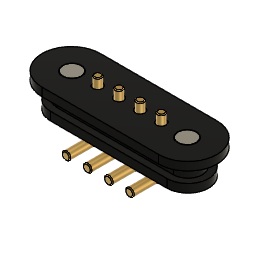
5358 Mag Connector (4-pin, Right Angle, Pins) (Autodesk Fusion 360 design; units mm, degrees)
Autodesk Fusion 360 part; units mm, degrees
sketch "Profile" plane through (0, 0, 0) normal (0, 0, 1) x (1, 0, 0)
  line L0 (0, 3.5) -> (0, -3.5) construction
  circle A0 centre (-6.91, 0) radius 1.125
  circle A1 centre (-3.81, 0) radius 0.45
  circle A2 centre (-1.27, 0) radius 0.45
  circle A3 centre (1.27, 0) radius 0.45
  circle A4 centre (6.91, 0) radius 1.125
  circle A5 centre (-3.81, 0) radius 0.5
  circle A6 centre (-3.81, 0) radius 0.9
  circle A7 centre (-1.27, 0) radius 0.5
  circle A8 centre (-1.27, 0) radius 0.9
  circle A9 centre (1.27, 0) radius 0.5
  circle A10 centre (1.27, 0) radius 0.9
  circle A11 centre (-3.81, 0) radius 0.575
  circle A12 centre (-1.27, 0) radius 0.575
  circle A13 centre (1.27, 0) radius 0.575
  line L1 (-10.5, 0) -> (10.5, 0) construction
  line L2 (-7, 1.725) -> (-7, -1.725) construction
  line L3 (-7, 2.5) -> (-7, -2.5) construction
  line L4 (-7, 3.5) -> (-7, -3.5) construction
  arc A14 (-7, 3.5) -> (-7, -3.5) centre (-7, 0) ccw
  arc A15 (-7, 1.725) -> (-7, -1.725) centre (-7, 0) ccw
  arc A16 (-7, 2.5) -> (-7, -2.5) centre (-7, 0) ccw
  line L5 (0, 3.5) -> (-7, 3.5)
  line L6 (0, -3.5) -> (-7, -3.5)
  line L7 (-7, 2.5) -> (0, 2.5)
  line L8 (-7, 1.725) -> (0, 1.725)
  line L9 (-7, -1.725) -> (0, -1.725)
  line L10 (-7, -2.5) -> (0, -2.5)
  circle A17 centre (3.81, 0) radius 0.45
  circle A18 centre (3.81, 0) radius 0.5
  circle A19 centre (3.81, 0) radius 0.9
  circle A20 centre (3.81, 0) radius 0.575
  line L11 (7, 1.725) -> (0, 1.725)
  line L12 (7, 2.5) -> (0, 2.5)
  line L13 (0, 3.5) -> (7, 3.5)
  arc A21 (7, -3.5) -> (7, 3.5) centre (7, 0) ccw
  arc A22 (7, -2.5) -> (7, 2.5) centre (7, 0) ccw
  arc A23 (7, -1.725) -> (7, 1.725) centre (7, 0) ccw
  line L14 (7, -1.725) -> (0, -1.725)
  line L15 (7, -2.5) -> (0, -2.5)
  line L16 (0, -3.5) -> (7, -3.5)
  line L17 (1, 3.375) -> (-1, 3.375)
  line L18 (1, 3.375) -> (1.875, 2.5)
  line L19 (-1, 3.375) -> (-1.875, 2.5)
  line L20 (1.25, 2.5) -> (1.25, 1.9)
  line L21 (1.25, 1.9) -> (-1.25, 1.9)
  line L22 (-1.25, 1.9) -> (-1.25, 2.5)
  dimension "d1" = 2.25
  dimension "d10" = 0.9
  dimension "d11" = 3.1
  dimension "d16" = 2.54
  dimension "d17" = 0
  dimension "d19" = 1
  dimension "d20" = 1.8
  dimension "d45" = 1.15
  dimension "d91" = 13.82
  dimension "d92" = 21
  dimension "d93" = 3.45
  dimension "d94" = 5
  dimension "d95" = 7
  dimension "d104" = 2
  dimension "d105" = 3.75
  dimension "d107" = 45
  dimension "d108" = 0.6
  dimension "d109" = 2.5
  constraint vertical L0
  constraint symmetric L0 A0 A4
  constraint concentric A1 A5
  constraint concentric A1 A6
  constraint midpoint origin L0
  constraint concentric A6 A11
  constraint horizontal L1
  constraint coincident A0.centre L1
  constraint coincident A1.centre L1
  constraint coincident L1 origin
  constraint midpoint L1 origin
  constraint perpendicular L1 L2
  constraint symmetric L1 L2.start L2.end
  constraint perpendicular L1 L3
  constraint symmetric L1 L3.start L3.end
  constraint vertical L4
  constraint symmetric L1 L4.start L4.end
  constraint midpoint L4 A14.centre
  constraint coincident L1.start A14
  constraint midpoint L2 A14.centre
  constraint midpoint L3 A14.centre
  constraint perpendicular L0 L5
  constraint perpendicular L0 L6
  constraint coincident L4.end A14.end
  constraint coincident A14 L4.start
  constraint collinear L2 L4
  constraint collinear L3 L4
  constraint coincident L0 L7.end
  constraint tangent A16 L7
  constraint coincident L0 L8.end
  constraint tangent A15 L8
  constraint coincident L0 L9.end
  constraint tangent A15 L9
  constraint coincident L0 L10.end
  constraint tangent A16 L10
  constraint symmetric L5.start L0 L13.start
  constraint symmetric L6.start L0 L16.start
  constraint symmetric L0 L2.start L11.start
  constraint symmetric L0 L2.end A23.start
  constraint symmetric L0 L3.start L12.start
  constraint symmetric L0 L3.end A22.start
  constraint symmetric L0 L4.start L13.end
  constraint symmetric L0 L4.end A21.start
  constraint symmetric L0 A14 A21
  constraint symmetric L0 A15 A23
  constraint symmetric L0 A16 A22
  constraint symmetric L0 L7.end L12.end
  constraint symmetric L0 L8.end L11.end
  constraint symmetric L0 L9.end L14.end
  constraint symmetric L0 L10.end L15.end
  constraint parallel L13 L17
  constraint symmetric L0 L17.start L17.end
  constraint coincident L12 L18.end
  constraint coincident L7 L19.end
  constraint symmetric L0 L18.end L19.end
  constraint coincident L12 L20.start
  constraint perpendicular L12 L20
  constraint perpendicular L20 L21
  constraint coincident L7 L22.end
  constraint perpendicular L7 L22
  constraint symmetric L0 L20.end L21.end
  measures "d1" diameter of A0
  measures "d10" diameter of A1
  measures "d11" distance of A0.centre A1.centre
  measures "d19" diameter of A5
  measures "d20" diameter of A6
  measures "d45" diameter of A11
  measures "d91" distance of A0.centre A4.centre
  measures "d92" distance of L1.start L1.end
  measures "d93" distance of L2.start L2.end
  measures "d94" distance of L3.start L3.end
  measures "d95" distance of L0.start L0.end
  measures "d104" distance of L17.start L17.end
  measures "d105" distance of L18.end L19.end
  measures "d107" angle of L17 L19
  measures "d108" distance of L20.start L20.end
  measures "d109" distance of L20.end L21.end
extrude "Extrude - Housing" add sketch "Profile" along normal blind 4 contours A15 L8 L9 L11 A23 L14 makes body 1
extrude "Extrude6" add sketch "Profile" against normal blind 1 from surface at 4 contours A14 L5 L6 L13 A21 L16 | A16 L7 L10 L12 A22 L15 L20 L21 L22 | L7 L12 L17 L18 L19 | L7 L12 L20 L21 L22 bodies 1
extrude "Extrude7" add sketch "Profile" against normal blind 0.65 from surface at 3 contours A16 L7 L10 L12 A22 L15 L20 L21 L22 | L7 L12 L20 L21 L22 bodies 1
extrude "Extrude8" add sketch "Profile" along normal blind 1 contours A16 L7 L10 L12 A22 L15 L20 L21 L22 | L7 L12 L20 L21 L22 bodies 1
extrude "Extrude - Housing Pin Clearance" add sketch "Profile" along normal up to surface (3.8 mm away) from surface at 0.2 contours A6 | A8 | A10 | A19 bodies 1
copy_body "Body->Comp1" bodies 1 removing the originals makes body 2 in component "Housing"
extrude "Extrude - Magnets" add sketch "Profile" along normal blind 4 separate body contours A0 | A4 makes body 3 at (-5.7906, -0.112, 1.3333) makes body 4 at (8.0336, -0.0561, 2.6667)
copy_body "Body->Comp2" bodies 3 removing the originals makes body 5 in component "Magnet"
fillet "Fillet - Magnets" radius 0.05 1 edges at (5.8611, -0.4068, 4) on bodies 4
fillet "Fillet1" radius 0.05 1 edges at (-7.9589, -0.4068, 4) on bodies 5 in component "Magnet"
fillet "Fillet2" radius 0.2 1 edges at (-7.9589, -0.4068, 0) on bodies 5 in component "Magnet"
fillet "Fillet3" radius 0.2 1 edges at (5.8611, -0.4068, 0) on bodies 4
copy_body "CutPasteBodies1" bodies 4 removing the originals makes body 6 in component "Magnet"
extrude "Extrude - Pin Bottom" add sketch "Profile" against normal blind 0.1 separate body contours A1 | A5 makes body 7 in component "Pins"
extrude "Extrude - Pin Base" add sketch "Profile" along normal blind 0.2 contours A1 | A5 | A6 | A11 bodies 7 in component "Pins"
extrude "Extrude - Pin Body" add sketch "Profile" along normal blind 3.6 contours A5 | A11 bodies 7 in component "Pins"
ref_plane "WorkPlane1" through (-2.54, 0, 0) normal (1, 0, 0) x (0, 1, 0)
sketch "Pin Right Angle Profile" plane through (-2.54, 0, 0) normal (1, 0, 0) x (0, 1, 0)
  line L0 (-2, 4) -> (2, 4)
  line L1 (-0.75, -1.4) -> (-3.85, -1.4)
  line L2 (0, 0) -> (0, -0.65)
  arc A0 (-0.75, -1.4) -> (0, -0.65) centre (-0.75, -0.65) ccw
  line L3 (-0.75, -0.65) -> (0, -0.65) construction
  line L4 (-0.75, -0.65) -> (-0.75, -1.4) construction
  line L5 (-2.1, 0.1) -> (-2.1, 1)
  dimension "d79" = 5.4
  dimension "d80" = 0.75
  dimension "d81" = 1.75
  constraint horizontal L1
  constraint coincident L2.start origin
  constraint vertical L2
  constraint coincident A0.centre L3.start
  constraint perpendicular L2 L3
  constraint perpendicular L3 L4
  constraint coincident L1.start A0.start
  measures "d79" distance of L0 L1
  measures "d80" distance of L2.end A0.centre
  measures "d81" distance of L1.end L5
sweep "Sweep - Pin Right Angle" add 1 faces at (-3.6297, -0.1824, -0.1) path "Pin Right Angle Profile" along L1 A0 L2 on bodies 7 bodies 7 in component "Pins"
fillet "Fillet - Pin" radius 0.1 1 edges at (-4.2762, -3.85, -1.5808) on bodies 7 in component "Pins"
pattern_linear "R-Pattern - Pins" count 4 spacing 2.54 along (1, 0, 0) of bodies 7 makes body 8 at (-0.6979, 0.0573, 1.3333) makes body 9 at (1.8421, 0.0573, 1.3333) makes body 10 at (4.3821, 0.0573, 1.3333) in component "Pins"
extrude "Extrude - Pin Contacts" add sketch "Profile" along normal blind 3.1 from surface at 2 separate body contours A1 makes body 11 in component "Pin Contacts"
fillet "Fillet - Contacts" radius 0.1 1 faces at (-3.6317, -0.0721, 5.1) on bodies 11 in component "Pin Contacts"
pattern_linear "R-Pattern - Contacts" count 4 spacing 2.54 along (1, 0, 0) of bodies 11 makes body 12 at (-0.8222, -0.0448, 3) makes body 13 at (1.7178, -0.0448, 3) makes body 14 at (4.2578, -0.0448, 3) in component "Pin Contacts"
extrude "Extrude1" add sketch "Profile" against normal blind 0.5 from surface at 3 contours L7 L12 L17 L18 L19 bodies 2 in component "Housing"
extrude "Extrude2" add sketch "Profile" against normal blind 0.5 contours L7 L12 L20 L21 L22 bodies 2 in component "Housing"
chamfer "Chamfer1" distance 0.3 distance2 0.5 1 edges at (0, 1.9, -0.5) measured on face at (-0.4167, 2.3, -0.5) on bodies 2 in component "Housing"
chamfer "Chamfer2" distance 0.2 distance2 0.5 2 edges at (-1.25, 2.35, -0.5) (1.25, 2.35, -0.5) measured on face at (-0.4167, 2.4, -0.5) measured on face at (-0.4167, 2.4, -0.5) on bodies 2 in component "Housing"
component "Housing" placed x (1, 0, 0) y (0, 1, 0) z (0, 0, 1) at (0, 0, 0)
component "Magnet" placed x (1, 0, 0) y (0, 1, 0) z (0, 0, 1) at (0, 0, 0)
component "Pins" placed x (1, 0, 0) y (0, 1, 0) z (0, 0, 1) at (0, 0, 0)
component "Pin Contacts" placed x (1, 0, 0) y (0, 1, 0) z (0, 0, 1) at (0, 0, 0)
equation "d14 = 4"
equation "d82 = -( ( 2.54 * 1 ) * 1 mm )"
equation "d91 = ( d11 * 2 ) + ( d16 * ( d14 - 1 ) )"
named bodies: "Housing", "Magnet", "Magnet (1)", "Magnet (2)", "Pin (1)", "Contact (1)", "Pin (2)", "Pin (3)", "Contact (2)", "Contact (3)", "Contact (1) (1)", "Pin (1) (1)"
